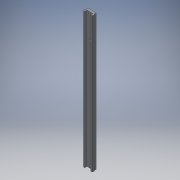
# Autodesk Inventor part: slider4b
Saved by Autodesk Inventor 2018.2 (Build 222227000, 227)
## iProperties
Created: 2018-02-09
Part Number: slider4b
Material: 一般
Document SubType Name: Modeling
Designer: SHUICHI
Density: 1 g/cm^3
Appearance: 既定
Author: SHUICHI
Autodesk Inventor part; units mm, degrees
ref_plane "YZ Plane" through (0, 0, 0) normal (1, 0, 0) x (0, 1, 0)
ref_plane "XZ Plane" through (0, 0, 0) normal (0, 1, 0) x (-1, 0, 0)
ref_plane "XY Plane" through (0, 0, 0) normal (0, 0, 1) x (1, 0, 0)
sketch "スケッチ1" plane through (0, 0, 0) normal (0, 0, 1) x (1, 0, 0)
  line L0 (0, 0) -> (16.2361, 0)
  line L1 (17, 8) -> (0, 8)
  line L2 (3, 0) -> (14, 0)
  line L3 (14, 0) -> (14, 4)
  line L4 (14, 4) -> (3, 4)
  line L5 (3, 4) -> (3, 0)
  arc A0 (16.2361, 0) -> (16, 4.2361) centre (14, 2) ccw
  arc A1 (1, 4.2361) -> (0.7639, 0) centre (3, 2) ccw
  line L6 (16, 8) -> (16, 4.2361)
  line L7 (1, 8) -> (1, 4.2361)
  point P0 (8.5, 8)
  point P1 (8.5, 4)
  dimension "d0" = 17
  dimension "d2" = 11
  dimension "d3" = 4
  dimension "d15" = 7.5
  dimension "d16" = 15
  dimension "d17" = 8
  dimension "d18" = 17
  constraints: 16 end point, 4 midpoint, 4 parallel, 4 point on circle, 4 point on line, 2 centre point, 2 horizontal, 2 perpendicular, 2 vertical alignment
  measures "d0" distance of L1.end L1.start
  measures "d2" distance of L4.end L3.end
  measures "d3" distance between parallel lines of L0 L4
  measures "d15" distance from line of point (8.5, 8) L7
  measures "d16" distance between parallel lines of L7 L6
  measures "d17" distance between parallel lines of L2 L1
extrude "押し出し1" add sketch "スケッチ1" along normal blind 246 contours A1 L7 L1 L6 A0 L0 L3 L4 L5
sketch "スケッチ2" plane through (0, 8, 0) normal (0, 1, 0) x (1, 0, 0)
  line L0 (16, 0) -> (0, 0) projected
  line L1 (-88, 0) -> (-88, -156.2142)
  line L2 (-88, -156.2142) -> (215.5, -300.2142)
  line L3 (3, 0) -> (3, -246) projected
  point P0 (8.5, -5)
  point P1 (8.5, -202)
  point P2 (8, 0)
  point P3 (17, 0)
  point P4 (1, 0)
  dimension "d6" = 5
  dimension "d20" = 96
  dimension "d21" = 303.5
  dimension "d22" = 144
  dimension "d23" = 5.5
  dimension "d24" = 197
  constraints: 4 end point, 1 horizontal alignment, 1 midpoint, 1 point on line, 1 vertical, 1 vertical alignment
  measures "d6" distance from line of L0 point (8.5, -5)
  measures "d20" distance from line of point (8, 0) L1
  measures "d21" horizontal distance of L1.end L2.end
  measures "d22" vertical distance of L1.end L2.end
  measures "d23" distance from line of point (8.5, -5) L3
  measures "d24" distance of point (8.5, -5) point (8.5, -202)
hole "穴1" at (8.5, 8, 5) at (8.5, 8, 202) direction (0, -1, 0) diameter 3 depth 8 tip angle 118
